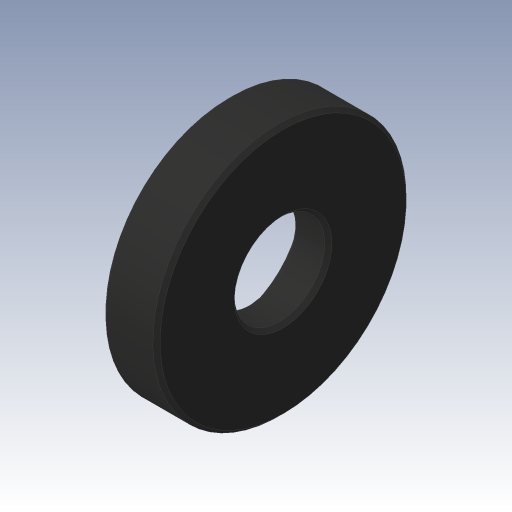
# Autodesk Inventor part: BT013_huenin20_23
Saved by Autodesk Inventor 2023.3 (Build 273359000, 359)
## iProperties
Company: HTBLA Kaindorf
RuleStatus: InUse
Created: 2023-12-01
Part Number: BT013_huenin20_23
Project: Fiberprinter-Hotend
Material: Gummi
Description: Faserführungsrad
Document SubType Name: Modeling
Designer: huenin20
Density: 0.93 g/cm^3
Appearance: Gummi - Schwarz
Mass: 0.343999 g
Surface Area: 4.43115 cm^2
Volume: 0.369891 cm^3
AfterDocNew0: iProperties-Editor_aufrufen
Author: nicob
Keywords: 2023
Autodesk Inventor part; units mm, degrees
ref_plane "YZ Plane" through (0, 0, 0) normal (1, 0, 0) x (0, 1, 0)
ref_plane "XZ Plane" through (0, 0, 0) normal (0, 1, 0) x (-1, 0, 0)
ref_plane "XY Plane" through (0, 0, 0) normal (0, 0, 1) x (1, 0, 0)
sketch "Skizze3" plane through (0, 0, 0) normal (1, 0, 0) x (0, 1, 0)
  line L0 (0, 0) -> (6.2939, 0)
  line L1 (0, 7) -> (0, 4)
  line L2 (0, 4) -> (1, 4)
  line L3 (1, 4) -> (1, 2.5)
  line L4 (1, 2.5) -> (3, 2.5)
  line L5 (3, 2.5) -> (3, 7)
  line L6 (3, 7) -> (0, 7)
  dimension "d4" = 14
  dimension "d5" = 5
  dimension "d6" = 3
  dimension "d7" = 1
  dimension "d9" = 8
  constraints: 14 end point, 5 perpendicular, 1 horizontal, 1 vertical, 1 vertical alignment
  measures "d4" diameter of L6 L0
  measures "d5" diameter of L4 L0
  measures "d6" distance of L5.end L1.start
  measures "d7" distance between parallel lines of L1 L3
  measures "d9" diameter of L2 L0
revolve "Umdrehung1" add sketch "Skizze3" angle 360 about axis through (0, 0, 0) along (0, 1, 0)
chamfer "Fase1" distance 0.2 angle 45 4 edges at (0, 3, -7) (0, 0, -7) (0, 3, -2.5) (0, 1, -2.5)
